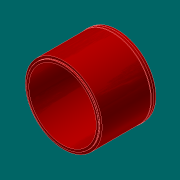
# Autodesk Inventor part: A1-19027-100-06 HCWI liner - pup
Saved by Autodesk Inventor 2017.3 (Build 213257000, 257)
## iProperties
Created: 2019-10-16
Part Number: A1-19027-100-06 HCWI liner - pup
Material: Iron, HCWI
Document SubType Name: Modeling
Designer: GVD
Density: 7.33517 g/cm^3
Appearance: Iron Gray(1)
Mass: 513799 g
Surface Area: 30363.9 cm^2
Volume: 70045.9 cm^3
Description: 28 1/2" ID x 2" WALL x 22 23/32" HCWI LINER PUP, ASTM A532 CLASS III TYPE A, PF# 470282
Author: GVD
Autodesk Inventor part; units mm, degrees
ref_plane "YZ Plane" through (0, 0, 0) normal (1, 0, 0) x (0, 1, 0)
ref_plane "XZ Plane" through (0, 0, 0) normal (0, 1, 0) x (-1, 0, 0)
ref_plane "XY Plane" through (0, 0, 0) normal (0, 0, 1) x (1, 0, 0)
sketch "Sketch1" plane through (0, 0, 0) normal (0, 0, 1) x (1, 0, 0)
  circle A0 centre (0, 0) radius 361.95
  circle A1 centre (0, 0) radius 412.75
  dimension "d0" = 723.9
  dimension "d1" = 825.5
  constraints: 2 centre point, 2 coincident
  measures "d0" diameter of A0
  measures "d1" diameter of A1
extrude "Extrusion1" add sketch "Sketch1" along normal blind 577
sketch "Sketch2" plane through (0, 0, 0) normal (0, 0, -1) x (-1, 0, 0)
  circle A0 centre (0, 0) radius 412.75 projected
  circle A1 centre (0, 0) radius 415.925
  dimension "d4" = 831.85
  constraints: 1 centre point, 1 coincident
  measures "d4" diameter of A1
extrude "Extrusion2" add sketch "Sketch2" against normal blind 50.8
sketch "Sketch3" plane through (0, 0, 0) normal (0, 0, -1) x (-1, 0, 0)
  circle A0 centre (0, 0) radius 415.925 projected
  circle A1 centre (0, 0) radius 412.496
  dimension "d7" = 824.992
  constraints: 1 centre point, 1 coincident
  measures "d7" diameter of A1
extrude "Extrusion3" cut sketch "Sketch3" against normal blind 25.4
chamfer "Chamfer1" distance 3.175 angle 45 1 edges at (-412.75, 0, 50.8)
sketch "Sketch4" plane through (0, 0, 577) normal (0, 0, 1) x (1, 0, 0)
  circle A0 centre (0, 0) radius 361.95 projected
  circle A1 centre (0, 0) radius 387.096
  dimension "d13" = 774.192
  constraints: 1 centre point, 1 coincident
  measures "d13" diameter of A1
extrude "Extrusion4" add sketch "Sketch4" along normal blind 12.7
fillet "Fillet1" radius 0.7937 2 edges at (-387.096, 0, 577) (412.496, 0, 25.4)
chamfer "Chamfer2" distance 0.7937 angle 45 1 edges at (-387.096, 0, 589.7)
equation "\"d10\" = -0.5 * d1 + 0.5 * d4"
body "Solid1"
